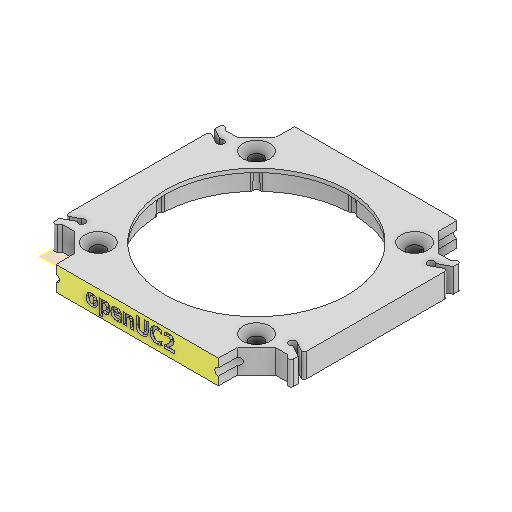
# Autodesk Inventor part: 10_Insert_v4
Saved by Autodesk Inventor 2025.1 (Build 291241020, 241B)
## iProperties
Created: 2024-08-17
Part Number: 10_Insert_v4
Material: Generisch
Document SubType Name: Modeling
Designer: diederichbenedict
Density: 1 g/cm^3
Appearance: Vorgabe
Author: diederichbenedict
Autodesk Inventor part; units mm, degrees
ref_plane "YZ Plane" through (0, 0, 0) normal (1, 0, 0) x (0, 1, 0)
ref_plane "XZ Plane" through (0, 0, 0) normal (0, 1, 0) x (-1, 0, 0)
ref_plane "XY Plane" through (0, 0, 0) normal (0, 0, 1) x (1, 0, 0)
ref_plane "Arbeitsebene1" through (-46.4439, 9.9695, -17) normal (0, 0, 1) x (1, 0, 0)
sketch "Skizze1" plane through (-46.4439, 9.9695, -17) normal (0, 0, 1) x (1, 0, 0)
  line L0 (0, -1.4142) -> (0, 34) projected
  line L1 (0, -1.4142) -> (1.4142, 0) projected
  line L2 (3.9, 0) -> (1.4142, 0) projected
  line L3 (3.9, 34) -> (3.9, 0) projected
  line L4 (0, 34) -> (3.9, 34) projected
  line L5 (7.9, -4) -> (3.9, 0) projected
  line L6 (7.9, -6.8036) -> (41.9, -6.8036) projected
  line L7 (41.9, -6.8036) -> (41.9, -4) projected
  line L8 (7.9, -4) -> (41.9, -4) projected
  line L9 (7.9, -6.8036) -> (7.9, -4) projected
  line L10 (7.9, -7.9) -> (7.9, -6.8036) projected
  line L11 (24.9, -6.8036) -> (24.9, 31.79)
  line L12 (7.9, -7.9) -> (24.9, -7.9)
  line L13 (24.9, -7.9) -> (24.9, -6.8036)
  line L14 (24.9, 17) -> (0, 17)
  line L15 (24.9, -4) -> (7.9, -4)
  line L16 (7.9, -4) -> (7.9, -7.9)
  line L17 (7.9, -7.9) -> (24.9, -7.9)
  line L18 (24.9, -7.9) -> (24.9, -4)
  point P0 (46.4439, -9.9695)
  dimension "d0" = 24.9
  constraints: 16 end point, 3 perpendicular, 3 point on line, 2 horizontal, 2 midpoint, 2 parallel, 1 vertical
  measures "d0" distance between parallel lines of L14 L12
extrude "Extrusion1" add sketch "Skizze1" along normal blind 5 contours L0 L14 L3 L2 L1 | L14 L11 L8 L5 L3 | L8 L11 L6 L9 | L6 L13 L12 L10
sketch "Skizze2" plane through (-46.4439, 9.9695, -12) normal (0, 0, 1) x (1, 0, 0)
  line L0 (24.9, -7.9) -> (24.9, 17) projected
  line L1 (24.9, 17) -> (0, 17) projected
  line L2 (0, 17) -> (0, -1.4142) projected
  line L3 (0, -1.4142) -> (1.4142, 0) projected
  line L4 (1.4142, 0) -> (3.9, 0) projected
  line L5 (3.9, 0) -> (7.9, -4) projected
  line L6 (7.9, -4) -> (7.9, -7.9) projected
  line L7 (7.9, -7.9) -> (24.9, -7.9) projected
  line L8 (7.9, -4) -> (7.9681, -7.9)
  line L9 (7.9, -7.9) -> (24.9, -7.9) projected
  line L10 (7.9, -4) -> (11.8006, -4) construction
  line L11 (0, 0.8079) -> (2.3543, 2.0839)
  line L12 (2.3543, 2.0839) -> (3.0288, 1.9381)
  line L13 (3.0288, 1.9381) -> (3.0288, 2.8858)
  line L14 (3.0288, 2.8858) -> (2.3543, 3.0316)
  line L15 (2.3543, 3.0316) -> (0, 1.7555)
  arc A0 (2.3543, 2.0839) -> (2.3543, 3.0316) centre (2.9262, 2.5578) ccw
  point P0 (46.4439, -9.9695)
  point P1 (7.9681, -7.9)
  dimension "d3" = 89
  constraints: 14 end point, 3 point on line, 2 parallel, 2 point on circle, 1 centre point, 1 equal length, 1 horizontal, 1 vertical
  measures "d3" angle of L8 L10
extrude "Extrusion2" cut sketch "Skizze2" against normal through all contours L7 L6 L8 | L15 L14 L13 L12 L11 L2 | A0 L12 L13 L14
fillet "Rundung1" radius 0.5 2 edges at (-46.4439, 8.5553, -14.5) (-46.4439, 11.7251, -14.5)
sketch "Skizze3" plane through (-21.5439, 2.0695, -17) normal (0, -1, 0) x (1, 0, 0)
  line L0 (-16.9319, 5) -> (-16.9319, 0) projected
  line L1 (-16.9319, 0) -> (0, 0) projected
  line L2 (0, 0) -> (0, 5) projected
  line L3 (-16.9319, 5) -> (0, 5) projected
  circle A0 centre (-16.9319, 2.5) radius 0.75
  point P0 (21.5439, 17)
  dimension "d7" = 1.5
  dimension "d10" = 2.5
  constraints: 1 centre point, 1 midpoint
  measures "d7" diameter of A0
  measures "d10" distance from line of A0.centre L3
extrude "Extrusion3" cut sketch "Skizze3" against normal blind 7 contours A0 L0 | L0 A0
mirror "Spiegeln1" about plane through (-21.5439, 26.9695, -17) normal (0, 1, 0) of "Extrusion1", "Extrusion2", "Rundung1", "Extrusion3"
mirror "Spiegeln2" about plane through (-21.5439, 2.0695, -17) normal (1, 0, 0) of "Extrusion1", "Extrusion2", "Rundung1", "Extrusion3", "Spiegeln1"
sketch "Skizze4" plane through (-46.4439, 9.9695, -12) normal (0, 0, 1) x (1, 0, 0)
  arc A0 (49.8, 31.4048) -> (49.0617, 31.8443) centre (49.3, 31.4048) ccw projected
  line L0 (49.0617, 31.8443) -> (47.4457, 30.9684) projected
  arc A1 (47.4457, 31.9161) -> (47.4457, 30.9684) centre (46.8738, 31.4422) ccw projected
  line L1 (47.4457, 31.9161) -> (49.8, 33.1921) projected
  line L2 (49.8, 34.2071) -> (49.8, 33.1921) projected
  arc A2 (49.8, 34.2071) -> (48.9464, 34.5607) centre (49.3, 34.2071) ccw projected
  line L3 (48.9464, 34.5607) -> (48.3858, 34) projected
  line L4 (48.3858, 34) -> (45.9, 34) projected
  line L5 (45.9, 34) -> (41.9, 38) projected
  line L6 (41.9, 38) -> (41.8319, 41.9) projected
  line L7 (41.8319, 41.9) -> (7.9681, 41.9) projected
  line L8 (7.9681, 41.9) -> (7.9, 38) projected
  line L9 (3.9, 34) -> (7.9, 38) projected
  line L10 (1.4142, 34) -> (3.9, 34) projected
  line L11 (0.8536, 34.5607) -> (1.4142, 34) projected
  arc A3 (0.8536, 34.5607) -> (0, 34.2071) centre (0.5, 34.2071) ccw projected
  line L12 (0, 33.1921) -> (0, 34.2071) projected
  line L13 (0, 33.1921) -> (2.3543, 31.9161) projected
  arc A4 (2.3543, 30.9684) -> (2.3543, 31.9161) centre (2.9262, 31.4422) ccw projected
  line L14 (2.3543, 30.9684) -> (0.7383, 31.8443) projected
  arc A5 (0.7383, 31.8443) -> (0, 31.4048) centre (0.5, 31.4048) ccw projected
  line L15 (0, 2.5952) -> (0, 31.4048) projected
  arc A6 (0, 2.5952) -> (0.7383, 2.1557) centre (0.5, 2.5952) ccw projected
  line L16 (0.7383, 2.1557) -> (2.3543, 3.0316) projected
  arc A7 (2.3543, 2.0839) -> (2.3543, 3.0316) centre (2.9262, 2.5578) ccw projected
  line L17 (2.3543, 2.0839) -> (0, 0.8079) projected
  line L18 (0, 0.8079) -> (0, -0.2071) projected
  arc A8 (0, -0.2071) -> (0.8536, -0.5607) centre (0.5, -0.2071) ccw projected
  line L19 (0.8536, -0.5607) -> (1.4142, 0) projected
  line L20 (1.4142, 0) -> (3.9, 0) projected
  line L21 (3.9, 0) -> (7.9, -4) projected
  line L22 (7.9, -4) -> (7.9681, -7.9) projected
  line L23 (7.9681, -7.9) -> (41.8319, -7.9) projected
  line L24 (41.8319, -7.9) -> (41.9, -4) projected
  line L25 (45.9, 0) -> (41.9, -4) projected
  line L26 (48.3858, 0) -> (45.9, 0) projected
  line L27 (48.9464, -0.5607) -> (48.3858, 0) projected
  arc A9 (48.9464, -0.5607) -> (49.8, -0.2071) centre (49.3, -0.2071) ccw projected
  line L28 (49.8, 0.8079) -> (49.8, -0.2071) projected
  line L29 (49.8, 0.8079) -> (47.4457, 2.0839) projected
  arc A10 (47.4457, 3.0316) -> (47.4457, 2.0839) centre (46.8738, 2.5578) ccw projected
  line L30 (47.4457, 3.0316) -> (49.0617, 2.1557) projected
  arc A11 (49.0617, 2.1557) -> (49.8, 2.5952) centre (49.3, 2.5952) ccw projected
  line L31 (49.8, 31.4048) -> (49.8, 2.5952) projected
  circle A12 centre (24.9, 17) radius 24.9
  circle A13 centre (24.9, 17) radius 20
  point P0 (46.4439, -9.9695)
  dimension "d15" = 40
  constraints: 3 tangent, 2 centre point, 1 coincident
  measures "d15" diameter of A13
extrude "Extrusion4" cut sketch "Skizze4" against normal through all contours A13
sketch "Skizze5" plane through (-46.4439, 9.9695, -12) normal (0, 0, 1) x (1, 0, 0)
  circle A0 centre (24.9, 17) radius 20 projected
  arc A1 (49.8, 31.4048) -> (49.0617, 31.8443) centre (49.3, 31.4048) ccw projected
  line L0 (49.0617, 31.8443) -> (47.4457, 30.9684) projected
  arc A2 (47.4457, 31.9161) -> (47.4457, 30.9684) centre (46.8738, 31.4422) ccw projected
  line L1 (47.4457, 31.9161) -> (49.8, 33.1921) projected
  line L2 (49.8, 34.2071) -> (49.8, 33.1921) projected
  arc A3 (49.8, 34.2071) -> (48.9464, 34.5607) centre (49.3, 34.2071) ccw projected
  line L3 (48.9464, 34.5607) -> (48.3858, 34) projected
  line L4 (48.3858, 34) -> (45.9, 34) projected
  line L5 (45.9, 34) -> (41.9, 38) projected
  line L6 (41.9, 38) -> (41.8319, 41.9) projected
  line L7 (41.8319, 41.9) -> (7.9681, 41.9) projected
  line L8 (7.9681, 41.9) -> (7.9, 38) projected
  line L9 (3.9, 34) -> (7.9, 38) projected
  line L10 (1.4142, 34) -> (3.9, 34) projected
  line L11 (0.8536, 34.5607) -> (1.4142, 34) projected
  arc A4 (0.8536, 34.5607) -> (0, 34.2071) centre (0.5, 34.2071) ccw projected
  line L12 (0, 33.1921) -> (0, 34.2071) projected
  line L13 (0, 33.1921) -> (2.3543, 31.9161) projected
  arc A5 (2.3543, 30.9684) -> (2.3543, 31.9161) centre (2.9262, 31.4422) ccw projected
  line L14 (2.3543, 30.9684) -> (0.7383, 31.8443) projected
  arc A6 (0.7383, 31.8443) -> (0, 31.4048) centre (0.5, 31.4048) ccw projected
  line L15 (0, 2.5952) -> (0, 31.4048) projected
  arc A7 (0, 2.5952) -> (0.7383, 2.1557) centre (0.5, 2.5952) ccw projected
  line L16 (0.7383, 2.1557) -> (2.3543, 3.0316) projected
  arc A8 (2.3543, 2.0839) -> (2.3543, 3.0316) centre (2.9262, 2.5578) ccw projected
  line L17 (2.3543, 2.0839) -> (0, 0.8079) projected
  line L18 (0, 0.8079) -> (0, -0.2071) projected
  arc A9 (0, -0.2071) -> (0.8536, -0.5607) centre (0.5, -0.2071) ccw projected
  line L19 (0.8536, -0.5607) -> (1.4142, 0) projected
  line L20 (1.4142, 0) -> (3.9, 0) projected
  line L21 (3.9, 0) -> (7.9, -4) projected
  line L22 (7.9, -4) -> (7.9681, -7.9) projected
  line L23 (7.9681, -7.9) -> (41.8319, -7.9) projected
  line L24 (41.8319, -7.9) -> (41.9, -4) projected
  line L25 (45.9, 0) -> (41.9, -4) projected
  line L26 (48.3858, 0) -> (45.9, 0) projected
  line L27 (48.9464, -0.5607) -> (48.3858, 0) projected
  arc A10 (48.9464, -0.5607) -> (49.8, -0.2071) centre (49.3, -0.2071) ccw projected
  line L28 (49.8, 0.8079) -> (49.8, -0.2071) projected
  line L29 (49.8, 0.8079) -> (47.4457, 2.0839) projected
  arc A11 (47.4457, 3.0316) -> (47.4457, 2.0839) centre (46.8738, 2.5578) ccw projected
  line L30 (47.4457, 3.0316) -> (49.0617, 2.1557) projected
  arc A12 (49.0617, 2.1557) -> (49.8, 2.5952) centre (49.3, 2.5952) ccw projected
  line L31 (49.8, 31.4048) -> (49.8, 2.5952) projected
  line L32 (41.4, 0.5) -> (8.4, 0.5)
  line L33 (8.4, 0.5) -> (8.4, 33.5)
  line L34 (8.4, 33.5) -> (41.4, 33.5)
  line L35 (41.4, 33.5) -> (41.4, 0.5)
  line L36 (41.4, 0.5) -> (8.4, 33.5) construction
  line L37 (8.4, 0.5) -> (41.4, 33.5) construction
  point P0 (46.4439, -9.9695)
  dimension "d18" = 33
  dimension "d19" = 33
  constraints: 12 end point, 2 midpoint, 2 parallel, 1 horizontal, 1 perpendicular
  measures "d18" distance of L33.end L34.end
  measures "d19" distance of L32.end L33.end
hole "Bohrung1" at (-38.0439, 43.4695, -12) at (-38.0439, 10.4695, -12) at (-5.0439, 43.4695, -12) at (-5.0439, 10.4695, -12) direction (0, 0, -1) diameter 2.8 end through all
sketch "Sketch6" plane through (-46.4439, 9.9695, -12) normal (0, 0, 1) x (1, 0, 0)
  circle A0 centre (24.9, 17) radius 20 projected
  circle A1 centre (24.9, 17) radius 19
  point P0 (46.4439, -9.9695)
  dimension "d27" = 1
  constraints: 1 centre point, 1 coincident
  measures "d27" radial gap between concentric circles of A0 A1
extrude "Extrusion5" add sketch "Sketch6" against normal blind 0.8
chamfer "Chamfer1" distance 1.4 angle 45 4 edges at (-5.0439, 44.8695, -12) (-5.0439, 11.8695, -12) (-38.0439, 11.8695, -12) (-38.0439, 44.8695, -12)
sketch "Sketch7" plane through (-46.4439, 9.9695, -17) normal (0, 0, -1) x (-1, 0, 0)
  circle A0 centre (-24.9, 17) radius 20 projected
  circle A1 centre (-24.9, -3) radius 0.5
  point P0 (-46.4439, -9.9695)
  point P1 (-25.4, -2.9938)
  point P2 (-24.4, -2.9938)
  dimension "d33" = 1
  constraints: 1 centre point, 2 other
  measures "d33" diameter of A1
extrude "Extrusion6" cut sketch "Sketch7" against normal up to surface (4.2 mm away)
fillet "Fillet2" radius 0.5 1 edges at (-22.0438, 6.9758, -14.9)
pattern_circular "Circular Pattern1" count 8 over 360 about axis through (-21.5439, 26.9695, -12) along (0, 0, -1) of "Extrusion6", "Fillet2"
sketch "Sketch8" plane through (-38.4758, 2.0695, -14.5) normal (0, -1, 0) x (1, 0, 0)
  line L0 (6.2, 1.7679) -> (27.9743, 1.7679) construction
  line L1 (27.9743, 1.7679) -> (27.9743, -2.7673) construction
  line L2 (27.9743, -2.7673) -> (6.2, -2.7673) construction
  line L3 (6.2, -2.7673) -> (6.2, 1.7679) construction
  spline S0 degree 2 poles (8.6408, -0.16) (8.6408, -0.7191) (8.0306, -1.3609) (7.4739, -1.3609) knots 0 0 0 1 2 2 2
  spline S1 degree 2 poles (7.4739, -1.3609) (6.9196, -1.3609) (6.3045, -0.7191) (6.3045, -0.16) knots 0 0 0 1 2 2 2
  spline S2 degree 2 poles (6.3045, -0.16) (6.3045, 0.4041) (6.9196, 1.0434) (7.4739, 1.0434) knots 0 0 0 1 2 2 2
  spline S3 degree 2 poles (7.4739, 1.0434) (8.0282, 1.0434) (8.6408, 0.4016) (8.6408, -0.16) knots 0 0 0 1 2 2 2
  spline S4 degree 2 poles (7.9188, -0.1648) (7.9188, 0.037) (7.8531, 0.3068) (7.7948, 0.387) knots 0 0 0 1 2 2 2
  spline S5 degree 2 poles (7.7948, 0.387) (7.7316, 0.4721) (7.5735, 0.5378) (7.4739, 0.5378) knots 0 0 0 1 2 2 2
  spline S6 degree 2 poles (7.4739, 0.5378) (7.3766, 0.5378) (7.2235, 0.4794) (7.1603, 0.3968) knots 0 0 0 1 2 2 2
  spline S7 degree 2 poles (7.1603, 0.3968) (7.0995, 0.319) (7.0265, 0.0443) (7.0265, -0.1648) knots 0 0 0 1 2 2 2
  spline S8 degree 2 poles (7.0265, -0.1648) (7.0265, -0.3715) (7.0946, -0.6267) (7.1505, -0.7045) knots 0 0 0 1 2 2 2
  spline S9 degree 2 poles (7.1505, -0.7045) (7.2064, -0.7823) (7.3766, -0.8553) (7.4787, -0.8553) knots 0 0 0 1 2 2 2
  spline S10 degree 2 poles (7.4787, -0.8553) (7.5638, -0.8553) (7.7389, -0.7823) (7.7923, -0.7094) knots 0 0 0 1 2 2 2
  spline S11 degree 2 poles (7.7923, -0.7094) (7.8531, -0.6243) (7.9188, -0.3788) (7.9188, -0.1648) knots 0 0 0 1 2 2 2
  spline S12 degree 2 poles (11.2324, -0.1284) (11.2324, -0.6705) (10.6829, -1.3342) (10.2794, -1.3342) knots 0 0 0 1 2 2 2
  spline S13 degree 2 poles (10.2794, -1.3342) (10.1116, -1.3342) (9.8612, -1.2588) (9.7202, -1.1762) knots 0 0 0 1 2 2 2
  line L4 (9.7202, -1.1762) -> (9.7202, -2.1194)
  line L5 (9.7202, -2.1194) -> (9.0152, -2.1194)
  line L6 (9.0152, -2.1194) -> (9.0152, 0.9729)
  line L7 (9.0152, 0.9729) -> (9.7202, 0.9729)
  line L8 (9.7202, 0.9729) -> (9.7202, 0.7347)
  spline S14 degree 2 poles (9.7202, 0.7347) (9.8758, 0.8684) (10.1967, 1.0337) (10.4082, 1.0337) knots 0 0 0 1 2 2 2
  spline S15 degree 2 poles (10.4082, 1.0337) (10.8021, 1.0337) (11.2324, 0.4089) (11.2324, -0.1284) knots 0 0 0 1 2 2 2
  spline S16 degree 2 poles (10.5103, -0.1429) (10.5103, 0.1877) (10.3061, 0.4843) (10.0922, 0.4843) knots 0 0 0 1 2 2 2
  spline S17 degree 2 poles (10.0922, 0.4843) (9.9974, 0.4843) (9.8102, 0.4235) (9.7202, 0.3627) knots 0 0 0 1 2 2 2
  line L9 (9.7202, 0.3627) -> (9.7202, -0.7726)
  spline S18 degree 2 poles (9.7202, -0.7726) (9.7761, -0.7969) (9.9123, -0.8164) (10.0047, -0.8164) knots 0 0 0 1 2 2 2
  spline S19 degree 2 poles (10.0047, -0.8164) (10.2599, -0.8164) (10.5103, -0.4809) (10.5103, -0.1429) knots 0 0 0 1 2 2 2
  spline S20 degree 2 poles (12.7713, -1.3512) (12.1295, -1.3512) (11.4463, -0.7386) (11.4463, -0.1721) knots 0 0 0 1 2 2 2
  spline S21 degree 2 poles (11.4463, -0.1721) (11.4463, 0.3822) (12.0833, 1.0434) (12.657, 1.0434) knots 0 0 0 1 2 2 2
  spline S22 degree 2 poles (12.657, 1.0434) (13.1748, 1.0434) (13.7, 0.4819) (13.7, -0.0384) knots 0 0 0 1 2 2 2
  line L10 (13.7, -0.0384) -> (13.7, -0.2937)
  line L11 (13.7, -0.2937) -> (12.1513, -0.2937)
  spline S23 degree 2 poles (12.1513, -0.2937) (12.1611, -0.4517) (12.2753, -0.6608) (12.3677, -0.724) knots 0 0 0 1 2 2 2
  spline S24 degree 2 poles (12.3677, -0.724) (12.4577, -0.7872) (12.7008, -0.8407) (12.8442, -0.8407) knots 0 0 0 1 2 2 2
  spline S25 degree 2 poles (12.8442, -0.8407) (12.9658, -0.8407) (13.204, -0.7872) (13.3037, -0.741) knots 0 0 0 1 2 2 2
  spline S26 degree 2 poles (13.3037, -0.741) (13.3912, -0.7045) (13.5371, -0.6146) (13.5833, -0.5805) knots 0 0 0 1 2 2 2
  line L12 (13.5833, -0.5805) -> (13.6586, -0.5805)
  line L13 (13.6586, -0.5805) -> (13.6586, -1.164)
  spline S27 degree 2 poles (13.6586, -1.164) (13.5711, -1.1981) (13.4301, -1.2564) (13.3037, -1.2856) knots 0 0 0 1 2 2 2
  spline S28 degree 2 poles (13.3037, -1.2856) (13.1894, -1.3172) (12.9463, -1.3512) (12.7713, -1.3512) knots 0 0 0 1 2 2 2
  spline S29 degree 2 poles (13.0047, 0.1318) (12.9998, 0.3554) (12.8029, 0.5913) (12.6011, 0.5913) knots 0 0 0 1 2 2 2
  spline S30 degree 2 poles (12.6011, 0.5913) (12.3945, 0.5913) (12.1611, 0.3433) (12.1489, 0.1318) knots 0 0 0 1 2 2 2
  line L14 (12.1489, 0.1318) -> (13.0047, 0.1318)
  line L15 (16.1797, -1.2904) -> (15.4698, -1.2904)
  line L16 (15.4698, -1.2904) -> (15.4698, -0.1697)
  spline S31 degree 2 poles (15.4698, -0.1697) (15.4698, -0.0311) (15.4479, 0.2412) (15.4188, 0.3044) knots 0 0 0 1 2 2 2
  spline S32 degree 2 poles (15.4188, 0.3044) (15.3823, 0.3822) (15.2462, 0.4478) (15.1295, 0.4478) knots 0 0 0 1 2 2 2
  spline S33 degree 2 poles (15.1295, 0.4478) (15.0444, 0.4478) (14.8669, 0.3822) (14.7672, 0.3117) knots 0 0 0 1 2 2 2
  line L17 (14.7672, 0.3117) -> (14.7672, -1.2904)
  line L18 (14.7672, -1.2904) -> (14.0622, -1.2904)
  line L19 (14.0622, -1.2904) -> (14.0622, 0.9729)
  line L20 (14.0622, 0.9729) -> (14.7672, 0.9729)
  line L21 (14.7672, 0.9729) -> (14.7672, 0.7225)
  spline S34 degree 2 poles (14.7672, 0.7225) (14.9398, 0.8684) (15.268, 1.0337) (15.4674, 1.0337) knots 0 0 0 1 2 2 2
  spline S35 degree 2 poles (15.4674, 1.0337) (15.8126, 1.0337) (16.1797, 0.5961) (16.1797, 0.1828) knots 0 0 0 1 2 2 2
  line L22 (16.1797, 0.1828) -> (16.1797, -1.2904)
  spline S36 degree 2 poles (17.9569, -1.3536) (17.3515, -1.3536) (16.7, -0.7702) (16.7, -0.2062) knots 0 0 0 1 2 2 2
  line L23 (16.7, -0.2062) -> (16.7, 1.7096)
  line L24 (16.7, 1.7096) -> (17.4536, 1.7096)
  line L25 (17.4536, 1.7096) -> (17.4536, -0.1624)
  spline S37 degree 2 poles (17.4536, -0.1624) (17.4536, -0.476) (17.6894, -0.7823) (17.9569, -0.7823) knots 0 0 0 1 2 2 2
  spline S38 degree 2 poles (17.9569, -0.7823) (18.217, -0.7823) (18.4601, -0.4882) (18.4601, -0.1624) knots 0 0 0 1 2 2 2
  line L26 (18.4601, -0.1624) -> (18.4601, 1.7096)
  line L27 (18.4601, 1.7096) -> (19.2137, 1.7096)
  line L28 (19.2137, 1.7096) -> (19.2137, -0.2037)
  spline S39 degree 2 poles (19.2137, -0.2037) (19.2137, -0.758) (18.5792, -1.3536) (17.9569, -1.3536) knots 0 0 0 1 2 2 2
  spline S40 degree 2 poles (21.0857, -1.3488) (20.4098, -1.3488) (19.6173, -0.5319) (19.6173, 0.2071) knots 0 0 0 1 2 2 2
  spline S41 degree 2 poles (19.6173, 0.2071) (19.6173, 0.9195) (20.4123, 1.7679) (21.0881, 1.7679) knots 0 0 0 1 2 2 2
  spline S42 degree 2 poles (21.0881, 1.7679) (21.2656, 1.7679) (21.5525, 1.7266) (21.6838, 1.6925) knots 0 0 0 1 2 2 2
  spline S43 degree 2 poles (21.6838, 1.6925) (21.7859, 1.6609) (22.0265, 1.5564) (22.1019, 1.5175) knots 0 0 0 1 2 2 2
  line L29 (22.1019, 1.5175) -> (22.1019, 0.8028)
  line L30 (22.1019, 0.8028) -> (22.0265, 0.8028)
  spline S44 degree 2 poles (22.0265, 0.8028) (21.9706, 0.8514) (21.8053, 0.9875) (21.7008, 1.0507) knots 0 0 0 1 2 2 2
  spline S45 degree 2 poles (21.7008, 1.0507) (21.5962, 1.1164) (21.3458, 1.2063) (21.2073, 1.2063) knots 0 0 0 1 2 2 2
  spline S46 degree 2 poles (21.2073, 1.2063) (21.0444, 1.2063) (20.7745, 1.1042) (20.6505, 0.9754) knots 0 0 0 1 2 2 2
  spline S47 degree 2 poles (20.6505, 0.9754) (20.5387, 0.8611) (20.3953, 0.4697) (20.3953, 0.2047) knots 0 0 0 1 2 2 2
  spline S48 degree 2 poles (20.3953, 0.2047) (20.3953, -0.0749) (20.5436, -0.4566) (20.6651, -0.5733) knots 0 0 0 1 2 2 2
  spline S49 degree 2 poles (20.6651, -0.5733) (20.7818, -0.6875) (21.0687, -0.7872) (21.2121, -0.7872) knots 0 0 0 1 2 2 2
  spline S50 degree 2 poles (21.2121, -0.7872) (21.3604, -0.7872) (21.6303, -0.6875) (21.7227, -0.6267) knots 0 0 0 1 2 2 2
  spline S51 degree 2 poles (21.7227, -0.6267) (21.8248, -0.566) (21.9779, -0.4371) (22.0338, -0.3861) knots 0 0 0 1 2 2 2
  line L31 (22.0338, -0.3861) -> (22.1019, -0.3861)
  line L32 (22.1019, -0.3861) -> (22.1019, -1.0911)
  spline S52 degree 2 poles (22.1019, -1.0911) (22.0192, -1.13) (21.8029, -1.2272) (21.6862, -1.2613) knots 0 0 0 1 2 2 2
  spline S53 degree 2 poles (21.6862, -1.2613) (21.5452, -1.305) (21.2996, -1.3488) (21.0857, -1.3488) knots 0 0 0 1 2 2 2
  line L33 (24.7445, -1.2904) -> (22.5395, -1.2904)
  line L34 (22.5395, -1.2904) -> (22.5395, -0.8018)
  spline S54 degree 2 poles (22.5395, -0.8018) (22.8191, -0.5781) (23.2664, -0.1843) (23.4342, -0.0068) knots 0 0 0 1 2 2 2
  spline S55 degree 2 poles (23.4342, -0.0068) (23.6554, 0.2242) (23.8523, 0.5767) (23.8523, 0.7614) knots 0 0 0 1 2 2 2
  spline S56 degree 2 poles (23.8523, 0.7614) (23.8523, 0.9705) (23.6019, 1.1942) (23.3782, 1.1942) knots 0 0 0 1 2 2 2
  spline S57 degree 2 poles (23.3782, 1.1942) (23.264, 1.1942) (23.0598, 1.1383) (22.9552, 1.0945) knots 0 0 0 1 2 2 2
  spline S58 degree 2 poles (22.9552, 1.0945) (22.8531, 1.0483) (22.7073, 0.9511) (22.6708, 0.9267) knots 0 0 0 1 2 2 2
  line L35 (22.6708, 0.9267) -> (22.6124, 0.9267)
  line L36 (22.6124, 0.9267) -> (22.6124, 1.5807)
  spline S59 degree 2 poles (22.6124, 1.5807) (22.7389, 1.6415) (23.2786, 1.7679) (23.529, 1.7679) knots 0 0 0 1 2 2 2
  spline S60 degree 2 poles (23.529, 1.7679) (24.0638, 1.7679) (24.6133, 1.2914) (24.6133, 0.8611) knots 0 0 0 1 2 2 2
  spline S61 degree 2 poles (24.6133, 0.8611) (24.6133, 0.5961) (24.3628, 0.0856) (24.0735, -0.2062) knots 0 0 0 1 2 2 2
  spline S62 degree 2 poles (24.0735, -0.2062) (23.8912, -0.3861) (23.5484, -0.6656) (23.4731, -0.724) knots 0 0 0 1 2 2 2
  line L37 (23.4731, -0.724) -> (24.7445, -0.724)
  line L38 (24.7445, -0.724) -> (24.7445, -1.2904)
  point P0 (38.4758, 14.5)
  constraints: 2 other
extrude "Extrusion7" cut sketch "Sketch8" against normal blind 0.5
sketch "Sketch9" plane through (-46.4439, 9.9695, -12.8) normal (0, 0, -1) x (-1, 0, 0)
  circle A0 centre (-24.9, 17) radius 19 projected
  arc A1 (-25.3383, -3.2406) -> (-25.7552, -2.9817) centre (-25.7766, -3.4813) ccw projected
  arc A2 (-25.3383, -3.2406) -> (-24.4617, -3.2406) centre (-24.9, -3) ccw projected
  arc A3 (-24.0448, -2.9817) -> (-24.4617, -3.2406) centre (-24.0234, -3.4813) ccw projected
  arc A4 (-24.0448, -2.9817) -> (-11.3755, 2.2661) centre (-24.9, 17) ccw projected
  arc A5 (-10.8976, 2.3778) -> (-11.3755, 2.2661) centre (-11.0374, 1.8977) ccw projected
  arc A6 (-10.8976, 2.3778) -> (-10.2778, 2.9976) centre (-10.7579, 2.8579) ccw projected
  arc A7 (-10.1661, 3.4755) -> (-10.2778, 2.9976) centre (-9.7977, 3.1374) ccw projected
  arc A8 (-10.1661, 3.4755) -> (-4.9183, 16.1448) centre (-24.9, 17) ccw projected
  arc A9 (-4.6594, 16.5617) -> (-4.9183, 16.1448) centre (-4.4188, 16.1234) ccw projected
  arc A10 (-4.6594, 16.5617) -> (-4.6594, 17.4383) centre (-4.9, 17) ccw projected
  arc A11 (-4.9183, 17.8552) -> (-4.6594, 17.4383) centre (-4.4188, 17.8766) ccw projected
  arc A12 (-4.9183, 17.8552) -> (-10.1661, 30.5245) centre (-24.9, 17) ccw projected
  arc A13 (-10.2778, 31.0024) -> (-10.1661, 30.5245) centre (-9.7977, 30.8626) ccw projected
  arc A14 (-10.2778, 31.0024) -> (-10.8976, 31.6222) centre (-10.7579, 31.1421) ccw projected
  arc A15 (-11.3755, 31.7339) -> (-10.8976, 31.6222) centre (-11.0374, 32.1023) ccw projected
  arc A16 (-11.3755, 31.7339) -> (-24.0448, 36.9817) centre (-24.9, 17) ccw projected
  arc A17 (-24.4617, 37.2406) -> (-24.0448, 36.9817) centre (-24.0234, 37.4812) ccw projected
  arc A18 (-24.4617, 37.2406) -> (-25.3383, 37.2406) centre (-24.9, 37) ccw projected
  arc A19 (-25.7552, 36.9817) -> (-25.3383, 37.2406) centre (-25.7766, 37.4812) ccw projected
  arc A20 (-25.7552, 36.9817) -> (-38.4245, 31.7339) centre (-24.9, 17) ccw projected
  arc A21 (-38.9024, 31.6222) -> (-38.4245, 31.7339) centre (-38.7626, 32.1023) ccw projected
  arc A22 (-38.9024, 31.6222) -> (-39.5222, 31.0024) centre (-39.0421, 31.1421) ccw projected
  arc A23 (-39.6339, 30.5245) -> (-39.5222, 31.0024) centre (-40.0023, 30.8626) ccw projected
  arc A24 (-39.6339, 30.5245) -> (-44.8817, 17.8552) centre (-24.9, 17) ccw projected
  arc A25 (-45.1406, 17.4383) -> (-44.8817, 17.8552) centre (-45.3813, 17.8766) ccw projected
  arc A26 (-45.1406, 17.4383) -> (-45.1406, 16.5617) centre (-44.9, 17) ccw projected
  arc A27 (-44.8817, 16.1448) -> (-45.1406, 16.5617) centre (-45.3813, 16.1234) ccw projected
  arc A28 (-44.8817, 16.1448) -> (-39.6339, 3.4755) centre (-24.9, 17) ccw projected
  arc A29 (-39.5222, 2.9976) -> (-39.6339, 3.4755) centre (-40.0023, 3.1374) ccw projected
  arc A30 (-39.5222, 2.9976) -> (-38.9024, 2.3778) centre (-39.0421, 2.8579) ccw projected
  arc A31 (-38.4245, 2.2661) -> (-38.9024, 2.3778) centre (-38.7626, 1.8977) ccw projected
  arc A32 (-38.4245, 2.2661) -> (-25.7552, -2.9817) centre (-24.9, 17) ccw projected
  point P0 (-46.4439, -9.9695)
extrude "Extrusion8" cut sketch "Sketch9" along normal through all draft 2 contours A0 | A1 A32 A31 A30 A29 A28 A27 A26 A25 A24 A23 A22 A21 A20 A19 A18 A17 A16 A15 A14 A13 A12 A11 A10 A9 A8 A7 A6 A5 A4 A3 A2
equation "\"d19\" = d18"
